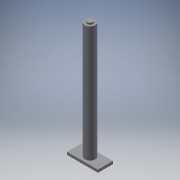
# Autodesk Inventor part: SyringeBody
Saved by Autodesk Inventor 2016 (Build 200138000, 138)
## iProperties
Created: 2017-02-19
Part Number: SyringeBody
Material: Generic
Document SubType Name: Modeling
Designer: Owner
Density: 1 g/cm^3
Appearance: Default
Author: Owner
Autodesk Inventor part; units mm, degrees
ref_plane "YZ Plane" through (0, 0, 0) normal (1, 0, 0) x (0, 1, 0)
ref_plane "XZ Plane" through (0, 0, 0) normal (0, 1, 0) x (-1, 0, 0)
ref_plane "XY Plane" through (0, 0, 0) normal (0, 0, 1) x (1, 0, 0)
sketch "Sketch1" plane through (0, 0, 0) normal (0, 1, 0) x (-1, 0, 0)
  circle A0 centre (0, 0) radius 3.275
  dimension "d0" = 6.55
  constraints: 1 centre point, 1 coincident
  measures "d0" diameter of A0
extrude "Extrusion1" add sketch "Sketch1" along normal blind 73.6
sketch "Sketch2" plane through (0, 0, 0) normal (0, -1, 0) x (1, 0, 0)
  circle A0 centre (0, 0) radius 1.9
  dimension "d3" = 3.8
  constraints: 1 centre point, 1 coincident
  measures "d3" diameter of A0
extrude "Extrusion2" cut sketch "Sketch2" against normal blind 70.8
sketch "Sketch3" plane through (0, 73.6, 0) normal (0, 1, 0) x (1, 0, 0)
  circle A0 centre (0, 0) radius 1.9
  constraints: 1 centre point, 1 coincident
extrude "Extrusion3" add sketch "Sketch3" along normal blind 1
sketch "Sketch4" plane through (0, 0, 0) normal (0, -1, 0) x (1, 0, 0)
  line L0 (0, 0) -> (0, 4.725)
  line L1 (0, 4.725) -> (0, -4.725)
  line L2 (0, 4.725) -> (9.75, 4.725)
  line L3 (9.75, 4.725) -> (-9.75, 4.725)
  line L4 (-9.75, 4.725) -> (-9.75, -4.725)
  line L5 (-9.75, -4.725) -> (9.75, -4.725)
  line L6 (9.75, -4.725) -> (9.75, 4.725)
  circle A0 centre (0, 0) radius 1.9 projected
  dimension "d8" = 4.725
  dimension "d9" = 9.45
  dimension "d10" = 9.75
  dimension "d11" = 19.5
  constraints: 14 end point, 3 perpendicular, 2 horizontal, 1 point on line, 1 vertical
  measures "d8" distance of L0.start L0.end
  measures "d9" distance of L0.end L1.end
  measures "d10" distance of L0.end L2.end
  measures "d11" distance of L2.end L3.end
extrude "Extrusion4" add sketch "Sketch4" along normal blind 1.75 contours A0 L1 L5 L4 L3 L0 | L0 L2 L6 L5 L1 A0
body "Solid1"
